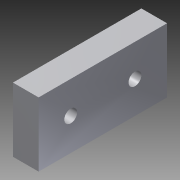
# Autodesk Inventor part: Leg_Link_Shim
Saved by Autodesk Inventor 2013 (Build 170138000, 138)
## iProperties
Created: 2014-04-20
Part Number: Leg_Link_Shim
Material: アセタール樹脂、白
Document SubType Name: Modeling
Designer: andou
Density: 1 g/cm^3
Author: andou
Autodesk Inventor part; units mm, degrees
ref_plane "YZ Plane" through (0, 0, 0) normal (1, 0, 0) x (0, 1, 0)
ref_plane "XZ Plane" through (0, 0, 0) normal (0, 1, 0) x (-1, 0, 0)
ref_plane "XY Plane" through (0, 0, 0) normal (0, 0, 1) x (1, 0, 0)
sketch "スケッチ1" plane through (0, 0, 0) normal (1, 0, 0) x (0, 1, 0)
  line L0 (-10, 5) -> (10, 5)
  line L1 (10, 5) -> (10, -5)
  line L2 (10, -5) -> (-10, -5)
  line L3 (-10, -5) -> (-10, 5)
  point P0 (0, 0)
  dimension "d0" = 20
  dimension "d2" = 10
  dimension "d3" = 10
  dimension "d4" = 5
  constraints: 8 end point, 2 parallel, 1 horizontal, 1 perpendicular
  measures "d0" distance of L0.start L0.end
  measures "d2" distance of L2.end L0.start
  measures "d3" distance from line of point (0, 0) L3
  measures "d4" distance from line of point (0, 0) L2
extrude "押し出し1" add sketch "スケッチ1" along normal blind 4
sketch "スケッチ2" plane through (4, 0, 0) normal (1, 0, 0) x (0, 0, -1)
  line L0 (5, -10) -> (5, 10) projected
  line L1 (5, 10) -> (-5, 10) projected
  circle A0 centre (0, 5) radius 1
  circle A1 centre (0, -5) radius 1
  point P0 (0, 0)
  dimension "d7" = 2
  dimension "d9" = 10
  dimension "d10" = 5
  dimension "d11" = 5
  dimension "d12" = 5
  constraints: 2 centre point, 1 equal radius
  measures "d7" diameter of A0
  measures "d9" distance of A1.centre A0.centre
  measures "d10" distance from line of L0 A1.centre
  measures "d11" distance from line of L0 A0.centre
  measures "d12" distance from line of L1 A0.centre
hole "穴1" at (4, 5, 0) at (4, -5, 0) direction (-1, 0, 0) diameter 2 end through all
